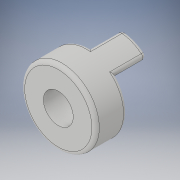
# Autodesk Inventor part: Flexible Shaft Coupling Iron Hub 1-4
Saved by Autodesk Inventor 2018 (Build 220112000, 112)
## iProperties
Created: 2020-03-23
Part Number: Flexible Shaft Coupling Iron Hub 1-4
Material: Generic
Document SubType Name: Modeling
Designer: emile
Density: 1 g/cm^3
Appearance: Default
Author: emile
Autodesk Inventor part; units mm, degrees
ref_plane "YZ Plane" through (0, 0, 0) normal (1, 0, 0) x (0, 1, 0)
ref_plane "XZ Plane" through (0, 0, 0) normal (0, 1, 0) x (-1, 0, 0)
ref_plane "XY Plane" through (0, 0, 0) normal (0, 0, 1) x (1, 0, 0)
sketch "Sketch1" plane through (0, 0, 0) normal (0, 0, 1) x (1, 0, 0)
  circle A0 centre (0, 0) radius 7.9375
  circle A1 centre (0, 0) radius 3.175
  line L0 (0, 7.9375) -> (0, 4.445)
  arc A2 (3.1431, 3.1431) -> (0, 4.445) centre (0, 0) ccw
  line L1 (3.1431, 3.1431) -> (5.6127, 5.6127)
  line L2 (0, 4.445) -> (0, 0) construction
  line L3 (0, 0) -> (3.1431, 3.1431) construction
  dimension "d0" = 15.875
  dimension "d1" = 6.35
  dimension "d2" = 45
  dimension "d3" = 1.27
  constraints: 8 end point, 4 point on circle, 3 centre point, 3 coincident, 2 collinear, 1 vertical
  measures "d0" diameter of A0
  measures "d1" diameter of A1
  measures "d2" angle of L1 L0
  measures "d3" radial gap between concentric circles of A1 A2
extrude "Extrusion1" add sketch "Sketch1" along normal blind 6.7469
extrude "Extrusion2" add sketch "Sketch1" against normal blind 6.7469 contours L1 A2 L0 A0 picked at (4.3885, 5.1185)
fillet "Fillet1" radius 0.7937 4 edges at (3.1431, 3.1431, -3.3734) (0, 4.445, -3.3734) (5.6127, 5.6127, -3.3734) (0, 7.9375, -3.3734)
pattern_circular "Circular Pattern1" count 2 over 360 about axis through (0, 0, 0) along (0, 0, 1) of "Extrusion2", "Fillet1"
fillet "Fillet2" radius 0.7937 21 edges at (0.0002, 7.9374, 0) (-7.6253, 2.2041, 0) (5.2917, 5.9163, 0) (7.1529, -3.4409, 0) (5.2514, 5.6255, -6.7469) (4.3409, 4.3409, -6.7469) (3.1606, 3.4314, -6.7469) (1.701, 4.1066, -6.7469) (0.1915, 4.6613, -6.7469) (0, 6.1389, -6.7469) (0.2646, 7.6911, -6.7469) (3.0375, 7.3333, -6.7469) (-5.6127, -5.6127, 6.7469) (-0.1915, -4.6613, -6.7469) (0, -6.1389, -6.7469) (-0.2646, -7.6911, -6.7469) (-3.0375, -7.3333, -6.7469) (-5.2514, -5.6255, -6.7469) (-4.3409, -4.3409, -6.7469) (-3.1606, -3.4314, -6.7469) (-1.701, -4.1066, -6.7469)
body "Solid1"
